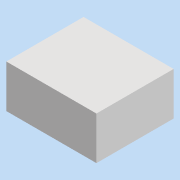
# Autodesk Inventor part: 22_Blocco_Escursione_Braccio
Saved by Autodesk Inventor 2020 (Build 240168000, 168)
## iProperties
Created: 2019-11-16
Part Number: 22_Blocco_Escursione_Braccio
Material: Generico
Document SubType Name: Modeling
Designer: socci
Density: 1 g/cm^3
Appearance: Default
Author: socci
Autodesk Inventor part; units mm, degrees
ref_plane "YZ Plane" through (0, 0, 0) normal (1, 0, 0) x (0, 1, 0)
ref_plane "XZ Plane" through (0, 0, 0) normal (0, 1, 0) x (-1, 0, 0)
ref_plane "XY Plane" through (0, 0, 0) normal (0, 0, 1) x (1, 0, 0)
sketch "Schizzo1" plane through (0, 0, 0) normal (0, 1, 0) x (-1, 0, 0)
  line L0 (5.2727, -129.2727) -> (-32.7273, -129.2727)
  line L1 (-32.7273, -129.2727) -> (-32.7273, -164.8727)
  line L2 (-32.7273, -164.8727) -> (5.2727, -164.8727)
  line L3 (5.2727, -164.8727) -> (5.2727, -129.2727)
  line L4 (5.2727, -129.2727) -> (-32.7273, -164.8727) construction
  line L5 (-32.7273, -129.2727) -> (5.2727, -164.8727) construction
  point P0 (0, 0)
  point P1 (-13.7273, -147.0727)
  dimension "d0" = 35.6
  dimension "d1" = 38
  constraints: 12 end point, 2 midpoint, 2 parallel, 1 horizontal, 1 perpendicular
  measures "d0" distance of L0.end L1.end
  measures "d1" distance of L0.start L0.end
extrude "Estrusione1" add sketch "Schizzo1" along normal blind 19.6
sketch "Schizzo2" plane through (0, 0, 0) normal (0, -1, 0) x (1, 0, 0)
  line L0 (-5.2727, -129.2727) -> (32.7273, -129.2727) projected
  line L1 (32.7273, -129.2727) -> (32.7273, -164.8727) projected
  line L2 (32.7273, -129.2727) -> (32.7273, -164.8727)
  line L3 (32.7273, -147.0727) -> (26.7273, -147.0727)
  line L4 (32.7273, -147.0727) -> (26.7273, -147.0727) construction
  line L5 (26.7273, -147.0727) -> (0.7273, -147.0727)
  line L6 (26.7273, -147.0727) -> (52.7273, -147.0727) construction
  point P0 (0, 0)
  dimension "d4" = 6
  dimension "d5" = 180
  dimension "d6" = 26
  dimension "d7" = 180
  constraints: 10 end point, 4 horizontal, 2 coincident, 2 collinear, 1 midpoint, 1 vertical
  measures "d4" distance of L3.start L3.end
  measures "d5" angle of L3 L4
  measures "d6" distance of L4.end L5.end
  measures "d7" angle of L5 L6
hole "Foro1" at (26.7273, 0, -147.0727) at (0.7273, 0, -147.0727) direction (0, 1, 0) diameter 5.9 end through all clearance for "Vite a testa piana" size "M5" standard "ANSI - Profilo M Metrico"
fillet "Raccordo1" radius 3 1 edges at (13.7273, 19.6, -129.2727)
fillet "Raccordo2" radius 3 1 edges at (13.7273, 19.6, -164.8727)
fillet "Raccordo3" radius 3 1 edges at (13.7273, 0, -164.8727)
fillet "Raccordo4" radius 3 1 edges at (13.7273, 0, -129.2727)
